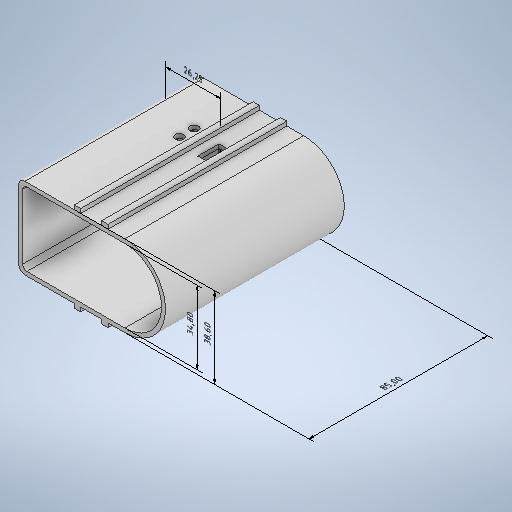
# Autodesk Inventor part: víko
Saved by Autodesk Inventor 2025.3 (Build 293356000, 356)
## iProperties
Created: 2025-06-12
Part Number: víko
Material: Generic
Document SubType Name: Modeling
Designer: Repete
Density: 1 g/cm^3
Appearance: Default
Author: Repete
Autodesk Inventor part; units mm, degrees
ref_plane "YZ Plane" through (0, 0, 0) normal (1, 0, 0) x (0, 1, 0)
ref_plane "XZ Plane" through (0, 0, 0) normal (0, 1, 0) x (-1, 0, 0)
sketch "Sketch1" plane through (0, 0, 0) normal (0, 1, 0) x (-1, 0, 0)
  line L0 (35.4, 17.4) -> (35.4, -17.4)
  line L1 (35.4, -17.4) -> (-13.2013, -17.4)
  arc A0 (-13.2013, 17.4) -> (-13.2013, -17.4) centre (-13.2013, 0) ccw
  line L2 (-13.2013, 17.4) -> (35.4, 17.4)
  line L3 (37.3, -19.3) -> (37.3, 19.3)
  line L4 (37.3, 19.3) -> (-13.2013, 19.3)
  arc A1 (-13.2013, 19.3) -> (-13.2013, -19.3) centre (-13.2013, 0) ccw
  line L5 (-13.2013, -19.3) -> (37.3, -19.3)
  point P0 (0, 0)
  point P1 (-13.2013, 0)
  point P2 (0, 0)
  point P3 (-12.8411, -36.7096)
  point P4 (-12.8411, -7.716)
  point P5 (-24.0253, -72.4098)
  constraints: 12 end point, 4 point on circle, 2 centre point, 2 parallel, 2 perpendicular
extrude "Extrusion1" add sketch "Sketch1" along normal blind 83
ref_plane "Work Plane1" through (0, 85, 0) normal (0, 1, 0) x (1, 0, 0)
sketch "Sketch2" plane through (0, 85, 0) normal (0, 1, 0) x (1, 0, 0)
  line L0 (-37.3, 19.3) -> (-37.3, -19.3)
  line L1 (-37.3, -19.3) -> (13.2013, -19.3)
  arc A0 (13.2013, -19.3) -> (13.2013, 19.3) centre (13.2013, 0) ccw
  line L2 (13.2013, 19.3) -> (-37.3, 19.3)
  point P0 (0, 0)
  point P1 (0, 0)
  point P2 (13.2013, 0)
  point P3 (0, 0)
  point P4 (14.0497, 95.3418)
  point P5 (14.0497, 124.3354)
  point P6 (2.8654, 59.6417)
  constraints: 6 end point, 2 point on circle, 1 centre point, 1 parallel, 1 perpendicular
extrude "Extrusion2" add sketch "Sketch2" against normal up to surface (2 mm away)
fillet "Fillet1" radius 3 3 edges at (-37.3, 41.5, -19.3) (-37.3, 84, -19.3) (-37.3, 42.5, 19.3)
fillet "Fillet2" radius 2 2 edges at (-35.4, 41.5, -17.4) (-35.4, 41.5, 17.4)
sketch "Sketch3" plane through (13.2013, 0, -19.3) normal (0, 0, -1) x (-1, 0, 0)
  line L0 (0, 85) -> (47.5013, 85) projected
  line L1 (0, 0) -> (47.5013, 0) projected
  line L2 (8, 85) -> (11, 85)
  line L3 (11, 85) -> (11, 0)
  line L4 (11, 0) -> (8, 0)
  line L5 (8, 0) -> (8, 85)
  line L6 (0, 0) -> (0, 85) projected
  point P0 (8, 0)
  point P1 (11, 85)
  dimension "d28" = 3
  dimension "d29" = 8
  constraints: 8 end point, 2 parallel, 2 point on line, 1 horizontal, 1 perpendicular
  measures "d28" distance between parallel lines of L5 L3
  measures "d29" distance between parallel lines of L6 L5
extrude "Extrusion5" add sketch "Sketch3" along normal blind 2 contours L0 L3 L1 L5
sketch "Sketch8" plane through (-34.3, 0, -19.3) normal (0, 0, -1) x (-1, 0, 0)
  line L0 (0, 85) -> (-47.5013, 85) projected
  line L1 (-36.5013, 0) -> (0, 0) projected
  line L2 (-26.5013, 85) -> (-23.5013, 85)
  line L3 (-23.5013, 85) -> (-23.5013, 0)
  line L4 (-23.5013, 0) -> (-26.5013, 0)
  line L5 (-26.5013, 0) -> (-26.5013, 85)
  line L6 (-36.5013, 0) -> (-36.5013, 85) projected
  point P0 (-34.3, 0)
  point P1 (-26.5013, 0)
  dimension "d34" = 10
  dimension "d35" = 3
  constraints: 8 end point, 2 parallel, 2 point on line, 1 horizontal, 1 perpendicular
  measures "d34" distance between parallel lines of L6 L5
  measures "d35" distance between parallel lines of L5 L3
extrude "Extrusion6" add sketch "Sketch8" along normal blind 2 contours L3 L1 L5 L0
sketch "Sketch9" plane through (13.2013, 0, 19.3) normal (0, 0, 1) x (1, 0, 0)
  line L0 (-47.5013, 85) -> (0, 85) projected
  line L1 (-46.6013, 0) -> (0, 0) projected
  line L2 (-11, 85) -> (-8, 85)
  line L3 (-8, 85) -> (-8, 0)
  line L4 (-8, 0) -> (-11, 0)
  line L5 (-11, 0) -> (-11, 85)
  line L6 (0, 0) -> (0, 85) projected
  point P0 (-13.2013, 0)
  point P1 (-11, 0)
  dimension "d38" = 8
  dimension "d39" = 3
  constraints: 8 end point, 2 parallel, 2 point on line, 1 horizontal, 1 perpendicular
  measures "d38" distance between parallel lines of L3 L6
  measures "d39" distance between parallel lines of L5 L3
extrude "Extrusion7" add sketch "Sketch9" along normal blind 2 contours L0 L3 L1 L5
sketch "Sketch10" plane through (-34.3, 0, 19.3) normal (0, 0, 1) x (1, 0, 0)
  line L0 (47.5013, 0) -> (0.9, 0) projected
  line L1 (23.5013, 85) -> (0, 85) projected
  line L2 (26.5013, 0) -> (23.5013, 0)
  line L3 (23.5013, 0) -> (23.5013, 85)
  line L4 (23.5013, 85) -> (26.5013, 85)
  line L5 (26.5013, 85) -> (26.5013, 0)
  line L6 (36.5013, 85) -> (36.5013, 0) projected
  point P0 (34.3, 0)
  point P1 (23.5013, 0)
  dimension "d42" = 10
  dimension "d43" = 3
  constraints: 8 end point, 2 parallel, 2 point on line, 1 horizontal, 1 perpendicular
  measures "d42" distance between parallel lines of L6 L5
  measures "d43" distance between parallel lines of L3 L5
extrude "Extrusion8" add sketch "Sketch10" along normal blind 2
sketch "Sketch14" plane through (13.2013, 83, 0) normal (0, -1, 0) x (1, 0, 0)
  line L0 (-46.6013, -17.4) -> (0, -17.4) projected
  line L1 (-45.348, -17.4) -> (-23.348, -17.4)
  line L2 (-23.348, -17.4) -> (-23.348, -2.4)
  line L3 (-23.348, -2.4) -> (-45.348, -2.4)
  line L4 (-45.348, -2.4) -> (-45.348, -17.4)
  line L5 (-46.348, -17.4) -> (-22.348, -17.4)
  line L6 (-22.348, -17.4) -> (-22.348, -1.4)
  line L7 (-22.348, -1.4) -> (-46.348, -1.4)
  line L8 (-46.348, -1.4) -> (-46.348, -17.4)
  point P0 (-13.2013, 0)
  point P1 (-23.348, -17.4)
  point P2 (-22.348, -17.4)
  dimension "d50" = 22
  dimension "d51" = 15
  dimension "d52" = 1
  dimension "d53" = 1
  dimension "d54" = 1
  constraints: 16 end point, 4 parallel, 2 horizontal, 2 perpendicular, 2 point on line
  measures "d50" distance of L2.end L3.end
  measures "d51" distance of L3.end L1.start
  measures "d52" distance between parallel lines of L3 L7
  measures "d53" distance between parallel lines of L4 L8
  measures "d54" distance between parallel lines of L6 L2
extrude "Extrusion11" add sketch "Sketch14" along normal blind 15 contours L8 L7 L6 L0 L2 L3 L4
sketch "Sketch16" plane through (-32.1466, 83, -17.4) normal (0, -1, 0) x (1, 0, 0)
  line L0 (0, 0) -> (22, 0)
  line L1 (22, 0) -> (22, 15)
  line L2 (22, 15) -> (0, 15)
  line L3 (0, 15) -> (0, 0)
  line L4 (0, 15) -> (22, 15) projected
  line L5 (22, 15) -> (22, 0) projected
  point P0 (32.1466, 17.4)
  dimension "d57" = 0
  dimension "d58" = 0
  constraints: 8 end point, 2 parallel, 1 horizontal, 1 perpendicular
  measures "d57" distance between parallel lines of L4 L2
  measures "d58" distance between parallel lines of L5 L1
extrude "Extrusion12" cut sketch "Sketch16" against normal through all
sketch "Sketch19" plane through (13.2013, 83, 0) normal (0, -1, 0) x (1, 0, 0)
  line L0 (0, 17.4) -> (-46.6013, 17.4) projected
  line L1 (-23.348, 17.4) -> (-45.348, 17.4)
  line L2 (-45.348, 17.4) -> (-45.348, 2.4)
  line L3 (-45.348, 2.4) -> (-23.348, 2.4)
  line L4 (-23.348, 2.4) -> (-23.348, 17.4)
  line L5 (-22.348, 17.4) -> (-46.348, 17.4)
  line L6 (-46.348, 17.4) -> (-46.348, 1.4)
  line L7 (-46.348, 1.4) -> (-22.348, 1.4)
  line L8 (-22.348, 1.4) -> (-22.348, 17.4)
  line L9 (-46.348, -1.4) -> (-46.348, -17.4) projected
  point P0 (-13.2013, 0)
  point P1 (-22.348, 9.4)
  dimension "d68" = 15
  dimension "d69" = 22
  dimension "d70" = 1
  dimension "d71" = 1
  dimension "d72" = 1
  dimension "d73" = 0
  constraints: 16 end point, 4 parallel, 2 horizontal, 2 perpendicular, 2 point on line, 1 midpoint
  measures "d68" distance between parallel lines of L1 L3
  measures "d69" distance between parallel lines of L4 L2
  measures "d70" distance between parallel lines of L3 L7
  measures "d71" distance between parallel lines of L2 L6
  measures "d72" distance from line of point (-22.348, 9.4) L4
  measures "d73" distance between parallel lines of L9 L6
extrude "Extrusion15" add sketch "Sketch19" along normal blind 15 contours L8 L7 L6 L0 L2 L3 L4
sketch "Sketch22" plane through (-32.1466, 83, 17.4) normal (0, -1, 0) x (1, 0, 0)
  line L0 (22, -15) -> (0, -15) projected
  line L1 (0, 0) -> (0, -15) projected
  line L2 (22, -15) -> (0, -15)
  line L3 (0, -15) -> (0, 0)
  line L4 (0, 0) -> (22, 0)
  line L5 (22, 0) -> (22, -15)
  point P0 (32.1466, -17.4)
  constraints: 8 end point, 2 parallel, 1 horizontal, 1 perpendicular
extrude "Extrusion16" cut sketch "Sketch22" against normal through all
sketch "Sketch28" plane through (2.2013, 0, 19.3) normal (0, 0, 1) x (1, 0, 0)
  line L0 (-5.75, 61.5) -> (-1.25, 61.5)
  line L1 (-1.25, 61.5) -> (-1.25, 51.5)
  line L2 (-1.25, 51.5) -> (-5.75, 51.5)
  line L3 (-5.75, 51.5) -> (-5.75, 61.5)
  line L4 (-10, 0) -> (0, 0) projected
  line L5 (11, 0) -> (11, 85) projected
  point P0 (-2.2013, 0)
  point P1 (-3.5, 61.5)
  point P2 (-3.5, 51.5)
  dimension "d106" = 61.5
  dimension "d107" = 10
  dimension "d108" = 4.5
  dimension "d109" = 12.25
  constraints: 8 end point, 2 midpoint, 2 parallel, 1 horizontal, 1 perpendicular
  measures "d106" distance between parallel lines of L4 L0
  measures "d107" distance of point (-3.5, 61.5) point (-3.5, 51.5)
  measures "d108" distance between parallel lines of L3 L1
  measures "d109" distance between parallel lines of L5 L1
extrude "Extrusion22" cut sketch "Sketch28" against normal up to surface (1.9 mm away)
sketch "Sketch31" plane through (-34.3, 0, 19.3) normal (0, 0, 1) x (1, 0, 0)
  line L0 (23.5013, 85) -> (23.5013, 0) projected
  line L1 (0, 85) -> (23.5013, 85) projected
  point P0 (34.3, 0)
  point P1 (18.5013, 62)
  dimension "d124" = 5
  dimension "d125" = 23
  measures "d124" distance from line of L0 point (18.501, 62)
  measures "d125" distance from line of L1 point (18.501, 62)
hole "Hole1" at (-15.7987, 62, 19.3) direction (0, 0, -1) diameter 4 depth 1.9
pattern_linear "Rectangular Pattern1" count 2 spacing 7 along (0, -1, 0) of "Hole1"
body "Solid1"
